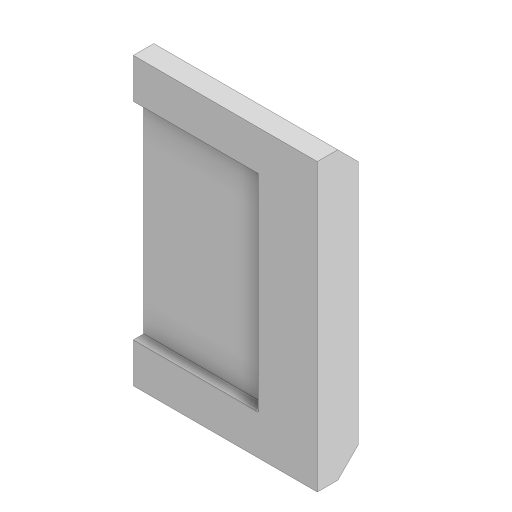
# Autodesk Inventor part: magnet_holder_ver.1
Saved by Autodesk Inventor 2024 (Build 280153000, 153)
## iProperties
Created: 2023-11-10
Part Number: magnet_holder_ver.1
Material: 一般
Document SubType Name: Modeling
Designer: moonshot
Density: 1 g/cm^3
Appearance: 既定
Author: moonshot
Autodesk Inventor part; units mm, degrees
ref_plane "YZ Plane" through (0, 0, 0) normal (1, 0, 0) x (0, 1, 0)
ref_plane "XZ Plane" through (0, 0, 0) normal (0, 1, 0) x (-1, 0, 0)
ref_plane "XY Plane" through (0, 0, 0) normal (0, 0, 1) x (1, 0, 0)
sketch "スケッチ1" plane through (0, 0, 0) normal (0, 0, 1) x (1, 0, 0)
  line L0 (-4.5, 7) -> (4.5, 7)
  line L1 (4.5, 7) -> (4.5, -7)
  line L2 (4.5, -7) -> (-4.5, -7)
  line L3 (-4.5, -7) -> (-4.5, 7)
  line L4 (0, -9.8) -> (0, 9.8) projected
  line L5 (-6.3, 0) -> (6.3, 0) projected
  point P0 (0, 0)
  dimension "d0" = 9
  dimension "d1" = 14
  constraints: 8 end point, 2 parallel, 1 horizontal, 1 perpendicular, 2 other
  measures "d0" distance of L0.start L0.end
  measures "d1" distance of L2.end L0.start
extrude "押し出し1" add sketch "スケッチ1" along normal mid plane 3
sketch "スケッチ2" plane through (0, 0, 1.5) normal (0, 0, 1) x (1, 0, 0)
  line L0 (-4.5, 7) -> (-4.5, -7) projected
  line L1 (-4.5, 5.05) -> (1.6, 5.05)
  line L2 (1.6, 5.05) -> (1.6, -5.05)
  line L3 (1.6, -5.05) -> (-4.5, -5.05)
  line L4 (-4.5, -5.05) -> (-4.5, 5.05)
  line L5 (-6.3, 0) -> (6.3, 0) projected
  point P0 (0, 0)
  dimension "d4" = 6.1
  dimension "d5" = 10.1
  constraints: 8 end point, 2 parallel, 1 horizontal, 1 perpendicular, 1 point on line, 1 other
  measures "d4" distance of L1.start L1.end
  measures "d5" distance of L1.end L2.end
extrude "押し出し2" cut sketch "スケッチ2" against normal blind 0.5
sketch "スケッチ3" plane through (0, 0, -1.5) normal (0, 0, -1) x (-1, 0, 0)
  circle A0 centre (0, 0) radius 1.5
  dimension "d8" = 3
  constraints: 1 centre point, 1 coincident
  measures "d8" diameter of A0
extrude "押し出し3" cut sketch "スケッチ3" against normal blind 0.5
chamfer "面取り1" distance 2 angle 45 2 edges at (0, -7, -1.5) (0, 7, -1.5)
chamfer "面取り2" distance 1 angle 45 1 edges at (4.5, 0, -1.5)
